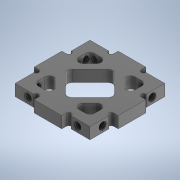
# Autodesk Inventor part: UpperArm_diagonal
Saved by Autodesk Inventor 2020 (Build 240168000, 168)
## iProperties
Created: 2021-09-07
Part Number: UpperArm_diagonal
Material: アセタール樹脂、黒
Document SubType Name: Modeling
Designer: aibay
Density: 1.425 g/cm^3
Appearance: 滑らか - 黒
Description: POM T5
Mass: 5.30964 g
Surface Area: 32.6127 cm^2
Volume: 3.72606 cm^3
Author: Masato Kubotera
Autodesk Inventor part; units mm, degrees
ref_plane "YZ Plane" through (0, 0, 0) normal (1, 0, 0) x (0, 1, 0)
ref_plane "XZ Plane" through (0, 0, 0) normal (0, 1, 0) x (-1, 0, 0)
ref_plane "XY Plane" through (0, 0, 0) normal (0, 0, 1) x (1, 0, 0)
sketch "スケッチ1" plane through (0, 0, 0) normal (0, 0, 1) x (1, 0, 0)
  line L0 (0, 16.25) -> (16.25, 16.25) construction
  line L1 (16.25, 16.25) -> (16.25, 0)
  line L2 (0, 0) -> (0, 16.25) construction
  line L3 (16.25, 16.25) -> (0, 0)
  line L4 (10.25, -2) -> (16.25, -2)
  line L5 (16.25, -2) -> (16.25, 0)
  line L6 (10.25, -2) -> (10.25, 0)
  arc A0 (10.25, 0) -> (8.15, 0) centre (9.2, 0) ccw
  line L7 (0, 0) -> (8.15, 0)
  line L8 (10.9467, 10.9467) -> (16.25, 5.6434)
  line L9 (4, 4) -> (13.6508, 4)
  line L10 (13.6508, 4) -> (8.8254, 8.8254)
  line L11 (4, 4) -> (4, 13.6508) construction
  arc A1 (4, 6) -> (6, 4) centre (6, 6) ccw
  point P0 (4.5858, 4.5858)
  dimension "d33" = 16.25
  dimension "d34" = 16.25
  dimension "d38" = 6
  dimension "d39" = 1.05
  dimension "d40" = 3
  dimension "d41" = 4
  dimension "d42" = 7.5
  dimension "d43" = 2
  dimension "d59" = 2
  constraints: 24 end point, 11 point on line, 5 perpendicular, 4 horizontal, 4 point on circle, 2 centre point, 2 tangent, 1 coincident, 1 parallel, 1 vertical
  measures "d33" distance of L0.start L0.end
  measures "d34" distance of L2.start L0.start
  measures "d38" distance of L4.start L4.end
  measures "d39" radius of A0
  measures "d40" distance between parallel lines of L10 L8
  measures "d41" distance between parallel lines of L7 L9
  measures "d42" distance from line of L8 L0.end
  measures "d43" distance of L4.start L6.end
  measures "d59" radius of A1
extrude "押し出し1" add sketch "スケッチ1" along normal blind 5 contours L1 L5 L4 L6 A0 L7 L3 L9 L10 L8 | A1 L9 L3
sketch "スケッチ2" plane through (8.15, 0, 0) normal (0, -1, 0) x (1, 0, 0)
  line L0 (-8.15, 0) -> (0, 0) projected
  line L1 (2.1, 0) -> (2.1, 5) projected
  line L2 (8.1, 0) -> (8.1, 5) projected
  point P0 (-2.65, 2.5)
  dimension "d46" = 2.5
  dimension "d56" = 10.75
  measures "d46" distance from line of L0 point (-2.65, 2.5)
  measures "d56" distance from line of L2 point (-2.65, 2.5)
hole "穴1" at (5.5, 0, 2.5) direction (0, 1, 0) diameter 3.242 depth 4 tip angle 118 thread size "M4x0.7" class "6H" standard "ISO Metric profile"
mirror "ミラー1" about plane through (16.25, -2, 0) normal (1, 0, 0) of "押し出し1", "穴1"
mirror "ミラー2" about plane through (21.5533, 10.9467, 0) normal (0.7071068, 0.7071068, 0) of "押し出し1", "穴1", "ミラー1"
mirror "ミラー3" about plane through (21.5533, 21.5533, 0) normal (-0.7071068, 0.7071068, 0) of "押し出し1", "穴1", "ミラー1", "ミラー2"
fillet "フィレット1" radius 2 12 edges at (13.6508, 4, 2.5) (4, 13.6508, 2.5) (16.25, 5.6434, 2.5) (5.6434, 16.25, 2.5) (16.25, 26.8566, 2.5) (26.8566, 16.25, 2.5) (28.5, 13.6508, 2.5) (28.5, 18.8492, 2.5) (13.6508, 28.5, 2.5) (4, 18.8492, 2.5) (18.8492, 4, 2.5) (18.8492, 28.5, 2.5)
equation "\"d34\" = d33"
